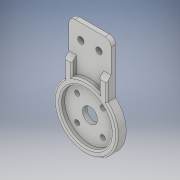
# Autodesk Inventor part: holder-LMF8LUU-z-axis
Saved by Autodesk Inventor 2018 (Build 220112000, 112)
## iProperties
Created: 2017-10-09
Part Number: holder-LMF8LUU-z-axis
Material: Generic
Document SubType Name: Modeling
Designer: Jurjen
Density: 1 g/cm^3
Appearance: Default
Author: Jurjen
Autodesk Inventor part; units mm, degrees
ref_plane "YZ Plane" through (0, 0, 0) normal (1, 0, 0) x (0, 1, 0)
ref_plane "XZ Plane" through (0, 0, 0) normal (0, 1, 0) x (-1, 0, 0)
ref_plane "XY Plane" through (0, 0, 0) normal (0, 0, 1) x (1, 0, 0)
sketch "Sketch1" plane through (0, 0, 0) normal (0, 0, 1) x (1, 0, 0)
  line L0 (-14, 17.1738) -> (14, 17.1738)
  line L1 (14, 17.1738) -> (14, -17.1738)
  line L2 (14, -32.8262) -> (-14, -32.8262)
  line L3 (-14, -32.8262) -> (-14, -17.1738)
  arc A0 (-14, -17.1738) -> (14, -17.1738) centre (0, -32.8262) ccw
  line L4 (-14, -17.1738) -> (-14, 17.1738)
  line L5 (14, -17.1738) -> (14, -32.8262)
  point P0 (0, 0)
  point P1 (0, 17.1738)
  point P2 (14, 0)
  dimension "d0" = 42
  dimension "d1" = 50
  dimension "d4" = 28
  constraints: 12 end point, 5 parallel, 3 midpoint, 2 horizontal alignment, 2 perpendicular, 2 point on circle, 2 vertical alignment, 1 centre point, 1 horizontal
  measures "d0" diameter of A0
  measures "d1" distance of L0.end L2.start
  measures "d4" distance between parallel lines of L1 L4
extrude "Extrusion1" add sketch "Sketch1" along normal blind 3
sketch "Sketch2" plane through (0, 0, 3) normal (0, 0, 1) x (1, 0, 0)
  line L0 (14, -17.1738) -> (14, 17.1738) projected
  line L1 (14, 17.1738) -> (-14, 17.1738) construction
  line L2 (-14, 17.1738) -> (-14, -17.1738) construction
  arc A0 (-14, -17.1738) -> (14, -17.1738) centre (0, -32.8262) ccw projected
  circle A1 centre (0, -32.8262) radius 16.75
  circle A2 centre (0, -32.8262) radius 21
  line L3 (-14, -2.8262) -> (14, -2.8262)
  line L4 (14, -17.1738) -> (14, 17.1738) construction
  line L5 (-14, 17.1738) -> (-14, -17.1738) projected
  line L6 (-14, -2.8262) -> (-14, -17.1738)
  line L7 (-9, -2.8262) -> (-9, -13.8526)
  line L8 (14, -2.8262) -> (14, -17.1738)
  line L9 (9, -13.8526) -> (9, -2.8262)
  arc A3 (-14, -17.1738) -> (14, -17.1738) centre (0, -32.8262) ccw projected
  line L10 (14, -2.8262) -> (14, -17.1738)
  point P0 (0, 0)
  dimension "d5" = 33.5
  dimension "d6" = 20
  dimension "d7" = 5
  dimension "d8" = 5
  constraints: 12 end point, 3 point on circle, 3 point on line, 2 centre point, 2 coincident, 2 collinear, 2 perpendicular, 2 vertical, 1 vertical alignment
  measures "d5" diameter of A1
  measures "d6" distance between parallel lines of L1 L3
  measures "d7" distance between parallel lines of L9 L0
  measures "d8" distance between parallel lines of L2 L7
extrude "Extrusion2" add sketch "Sketch2" along normal blind 3 contours A2 L9 L3 L0 | A0 A2 | L5 L3 L7 A2
sketch "Sketch3" plane through (0, 0, 3) normal (0, 0, 1) x (1, 0, 0)
  circle A0 centre (0, -32.8262) radius 16.75 projected
  circle A1 centre (0, -32.8262) radius 5
  line L0 (9, -2.8262) -> (14, -2.8262) projected
  line L1 (14, -2.8262) -> (14, 17.1738) projected
  line L2 (14, 17.1738) -> (-14, 17.1738) projected
  line L3 (-14, 17.1738) -> (-14, -2.8262) projected
  line L4 (-14, -2.8262) -> (-9, -2.8262) projected
  line L5 (-9, -2.8262) -> (-9, -13.8526) projected
  arc A2 (9, -13.8526) -> (-9, -13.8526) centre (0, -32.8262) ccw projected
  line L6 (9, -13.8526) -> (9, -2.8262) projected
  circle A3 centre (-6, 7.1738) radius 2.1
  circle A4 centre (6, 7.1738) radius 2.1
  line L7 (-6, 7.1738) -> (6, 7.1738) construction
  point P0 (0, 0)
  point P1 (0, 7.1738)
  dimension "d11" = 10
  dimension "d12" = 4.2
  dimension "d13" = 12
  dimension "d14" = 10
  constraints: 3 centre point, 2 end point, 1 coincident, 1 equal radius, 1 horizontal, 1 midpoint, 1 vertical alignment
  measures "d11" diameter of A1
  measures "d12" diameter of A3
  measures "d13" distance of L7.end L7.start
  measures "d14" distance between parallel lines of L2 L7
extrude "Extrusion3" cut sketch "Sketch3" against normal up to next contours A1 | A3 | A4
chamfer "Chamfer1" distance 3 angle 45 2 edges at (11.5, -2.8262, 6) (-11.5, -2.8262, 6)
fillet "Fillet1" radius 1 7 edges at (-16.75, -32.8262, 6) (0, -11.8262, 6) (0, -53.8262, 6) (-14, -11.4998, 6) (-9, -9.8392, 6) (9, -9.8392, 6) (14, -11.4998, 6)
sketch "Sketch4" plane through (0, -32.8262, 3) normal (0, 0, 1) x (1, 0, 0)
  circle A0 centre (0, 0) radius 5 projected
  circle A1 centre (8.4853, 8.4853) radius 1.65
  line L0 (0, 0) -> (8.4853, 8.4853) construction
  line L1 (0, 0) -> (0, 12.1192) construction
  line L2 (0, 0) -> (-12.1192, 0) construction
  circle A2 centre (-8.4853, 8.4853) radius 1.65
  line L3 (0, 0) -> (0, -12.1192) construction
  circle A3 centre (-8.4853, -8.4853) radius 1.65
  line L4 (0, 0) -> (12.1192, 0) construction
  circle A4 centre (8.4853, -8.4853) radius 1.65
  point P0 (0, 32.8262)
  dimension "d21" = 45
  dimension "d22" = 3.3
  dimension "d23" = 12
  dimension "d26" = 360
  constraints: 10 end point, 4 centre point, 2 coincident, 1 vertical, 19 other
  measures "d21" angle of L1 L0
  measures "d22" diameter of A1
  measures "d23" distance of L0.start L0.end
extrude "Extrusion4" cut sketch "Sketch4" against normal up to next contours A1 | A2 | A3 | A4
fillet "Fillet2" radius 4 2 edges at (-14, 17.1738, 1.5) (14, 17.1738, 1.5)
equation "\"d8\" = d7"
body "Solid1"
